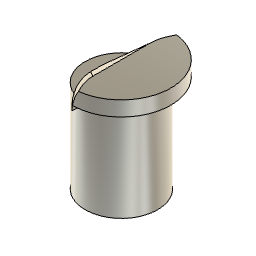
Pin for limit switch holder (Autodesk Fusion 360 design; units mm, degrees)
Autodesk Fusion 360 part; units mm, degrees
sketch "Sketch1" plane through (0, 0, 0) normal (0, 0, 1) x (1, 0, 0)
  circle A0 centre (0, 0) radius 5.5
  dimension "d1" = 11
  constraint coincident A0.centre origin
  measures "d1" diameter of A0
extrude "Extrude1" add sketch "Sketch1" along normal blind 14 contours A0 picked at (-1.490696, 0.273244)
sketch "Sketch2" plane through (0, 0, 14) normal (0, 0, 1) x (-1, 0, 0)
  circle A0 centre (0, 0) radius 5.5
  arc A1 (0, 7.5) -> (0, -7.5) centre (0, 0) ccw
  line L0 (0, 0) -> (0, -7.5)
  line L1 (0, 7.5) -> (0, 0)
  line L2 (0, 7.5) -> (3.739281, 4.033333)
  line L3 (0, -7.5) -> (3.739281, -4.033333)
  line L4 (3.739281, 4.033333) -> (3.739281, -4.033333)
  dimension "d8" = 7.5
  constraint coincident A0.centre A1.centre
  constraint vertical L0
  constraint parallel L0 L1
  constraint tangent A0 L2
  constraint tangent A0 L3
  measures "d8" radius of A1
extrude "Extrude3" add sketch "Sketch2" along normal blind 3 contours A0 L0 L1 L4 | A0 L1 L2 | A0 L0 L3 picked at (2.492854, 0) picked at (0.273094, 6.146212) picked at (0.273094, -6.146212)
extrude "Extrude4" add sketch "Sketch2" along normal blind 3 contours A0 L0 L1 | A0 A1 L0 L1 picked at (-2.680341, 2.486993) picked at (-1.649878, -6.612893)
chamfer "Chamfer1" distance 3.75 distance2 3 1 edges at (-3.739281, 0, 17) measured on face at (0.000156, 0.186825, 17)
fillet "Fillet1" radius 4 2 edges at (-1.86964, 5.766667, 15.495712) (-1.86964, -5.766667, 15.495712)
extrude "Extrude5" cut sketch "Sketch2" along normal blind 0.75 contours A0 A1 L0 L1 picked at (-1.649878, -6.612893)
equation "d8 = 5.500 mm + 2 mm"
